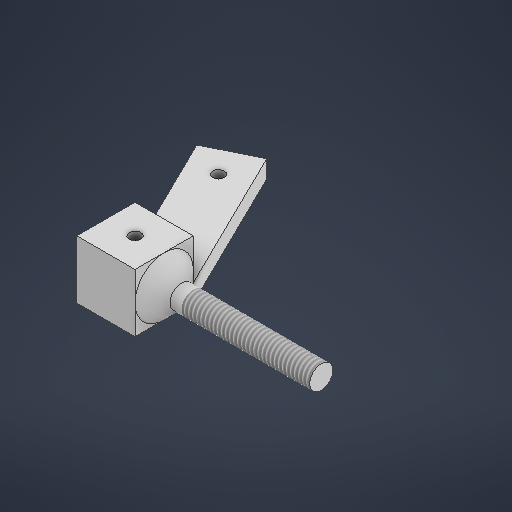
# Autodesk Inventor part: Front_Wheel_Anchor
Saved by Autodesk Inventor 2025 (Build 290162010, 162A)
## iProperties
Created: 2024-05-20
Part Number: Front_Wheel_Anchor
Material: Generic
Document SubType Name: Modeling
Designer: Garfieldcmix
Density: 1 g/cm^3
Appearance: Default
Author: Garfieldcmix
Autodesk Inventor part; units mm, degrees
ref_plane "YZ Plane" through (0, 0, 0) normal (1, 0, 0) x (0, 1, 0)
ref_plane "XZ Plane" through (0, 0, 0) normal (0, 1, 0) x (-1, 0, 0)
ref_plane "XY Plane" through (0, 0, 0) normal (0, 0, 1) x (1, 0, 0)
derived "Car_Plan.ipt"
sketch "Car_Sketch" plane through (0, 0, 0) normal (0, 1, 0) x (-1, 0, 0)
  line L0 (0, 0) -> (94, 0)
  line L1 (0, 0) -> (0, 105)
  line L2 (94, 0) -> (94, 105)
  line L3 (0, 105) -> (20, 105)
  line L4 (20, 105) -> (20, 190)
  line L5 (20, 190) -> (74, 190)
  line L6 (74, 190) -> (74, 105)
  line L7 (74, 105) -> (94, 105)
  line L8 (-5, 68) -> (-5, 0)
  line L9 (-5, 0) -> (-32, 0)
  line L10 (-32, 0) -> (-32, 68)
  line L11 (-32, 68) -> (-5, 68)
  line L12 (47, 190) -> (47, 0) construction
  line L13 (126, 68) -> (99, 68)
  line L14 (99, 68) -> (99, 0)
  line L15 (126, 0) -> (126, 68)
  line L16 (99, 0) -> (126, 0)
  line L17 (-5, 34) -> (99, 34) construction
  line L18 (0, 95) -> (94, 95) construction
  line L19 (-5, 190) -> (-32, 190)
  line L20 (-32, 122) -> (-5, 122)
  line L21 (-32, 190) -> (-32, 122)
  line L22 (-5, 122) -> (-5, 190)
  line L23 (-5, 156) -> (99, 156) construction
  line L24 (126, 122) -> (99, 122)
  line L25 (126, 190) -> (126, 122)
  line L26 (99, 190) -> (126, 190)
  line L27 (99, 122) -> (99, 190)
  line L28 (0, 156) -> (47, 34) construction
  line L29 (94, 156) -> (47, 34) construction
  line L30 (0, 156) -> (-174.2341, 34) construction
  line L31 (-5, 34) -> (-174.2341, 34) construction
  line L32 (8.9873, 132.6713) -> (47, 141.55) construction
  line L33 (85.0127, 132.6713) -> (47, 141.55) construction
sketch "Base" plane through (0, 0, 0) normal (0, 1, 0) x (-1, 0, 0)
  line L0 (-5, 161) -> (5, 161)
  line L1 (5, 161) -> (5, 151)
  line L2 (5, 151) -> (-5, 151)
  line L3 (-5, 151) -> (-5, 161)
  line L4 (-5, 156) -> (99, 156) construction
  line L5 (5, 151) -> (15.2194, 130.1584)
  line L6 (15.2194, 130.1584) -> (7.1577, 126.2055)
  line L7 (7.1577, 126.2055) -> (-5, 151)
  line L8 (8.9873, 132.6713) -> (13.0181, 134.6478) construction
  line L9 (8.9873, 132.6713) -> (4.9564, 130.6948) construction
  circle A0 centre (0, 156) radius 1
  circle A1 centre (8.9873, 132.6713) radius 1
  point P0 (0, 0)
  point P1 (11.1886, 128.1819)
  dimension "d187" = 10
  dimension "d189" = 10
  dimension "d190" = 5
  dimension "d191" = 5
  dimension "d194" = 5
  dimension "d199" = 2
  dimension "d200" = 2
  constraints: 18 end point, 4 perpendicular, 3 parallel, 2 centre point, 2 coincident, 2 collinear, 2 point on line, 1 midpoint
  measures "d187" distance of L0.start L0.end
  measures "d189" distance of L1.end L0.end
  measures "d190" distance from line of L0 point (0, 156)
  measures "d191" distance from line of L1 point (0, 156)
  measures "d194" distance of point (11.189, 128.182) L8.start
  measures "d199" diameter of A0
  measures "d200" diameter of A1
extrude "Anchor_Extrusion" add sketch "Base" along normal blind 10 contours L0 L1 L2 L3
extrude "Ackerman_Extrusion" add sketch "Base" along normal blind 3 contours L2 L5 L6 L7
sketch "Wheel_Screw" plane through (5, 0, 161) normal (1, 0, 0) x (0, 0, -1)
  line L0 (0, 0) -> (10, 0) projected
  line L1 (0, 0) -> (0, 10) projected
  line L2 (0, 10) -> (10, 10) projected
  line L3 (10, 3) -> (10, 10) projected
  line L4 (10, 0) -> (10, 3) projected
  circle A0 centre (5, 5) radius 2
  line L5 (10, 10) -> (0, 10) projected
  point P0 (161, 0)
  point P1 (5, 10)
  point P2 (0, 5)
  dimension "d201" = 4
  dimension "d202" = 5
  dimension "d203" = 5
  constraints: 2 midpoint, 1 centre point
  measures "d201" diameter of A0
  measures "d202" distance of point (5, 10) A0.centre
  measures "d203" distance of point (0, 5) A0.centre
extrude "Wheel_Screw_Extrusion" add sketch "Wheel_Screw" along normal blind 27 contours A0
chamfer "Chamfer7" distance 3 angle 45 1 edges at (5, 5, 158)
thread "Thread3" size "M4x0.7" class "6g" standard "ANSI Metric M Profile" length 22 offset 2
body "Solid4"
